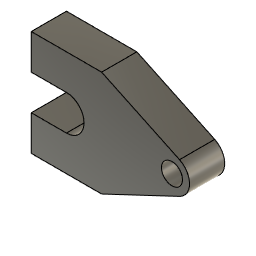
Part 9 (Autodesk Fusion 360 design; units mm, degrees)
Autodesk Fusion 360 part; units mm, degrees
sketch "Sketch2" plane through (0, 0, 0) normal (0, 1, 0) x (1, 0, 0)
  line L0 (-80, 30) -> (-40, 30)
  line L1 (-40, 30) -> (4.2788, 9.0384)
  arc A0 (4.2788, -9.0384) -> (4.2788, 9.0384) centre (0, 0) ccw
  line L2 (4.2788, -9.0384) -> (-40, -30)
  line L3 (-40, -30) -> (-80, -30)
  circle A1 centre (0, 0) radius 6
  line L4 (-80, -10) -> (-60, -10)
  arc A2 (-60, -10) -> (-60, 10) centre (-60, 0) ccw
  line L5 (-60, 10) -> (-80, 10)
  line L6 (-80, -30) -> (-80, -10)
  line L7 (-80, 10) -> (-80, 30)
  line L8 (0, 0) -> (-89, 0) construction
  dimension "d22" = 12
  dimension "d23" = 10
  dimension "d24" = 20
  dimension "d25" = 20
  dimension "d26" = 40
  dimension "d27" = 60
  dimension "d28" = 80
  dimension "d29" = 10
  constraint horizontal L0
  constraint tangent L1 A0
  constraint tangent A0 L2
  constraint parallel L0 L3
  constraint perpendicular L0 L6
  constraint concentric A0 A1
  constraint coincident A0.centre A1.centre
  constraint perpendicular L4 L6
  constraint tangent L4 A2
  constraint coincident L5.end L6
  constraint tangent A2 L5
  constraint perpendicular L5 L6
  constraint collinear L6 L7
  constraint horizontal L8
  constraint coincident A2.centre L8
  constraint equal L6 L7
  constraint equal L0 L3
  measures "d22" diameter of A1
  measures "d23" radius of A2
  measures "d24" distance of L3.end L4.start
  measures "d25" distance of A2.centre L7
  measures "d26" distance of L0.start L0.end
  measures "d27" distance of L0 L3
  measures "d28" distance of A0.centre L7
  measures "d29" radius of A0
extrude "Extrude2" add sketch "Sketch2" along normal blind 20
